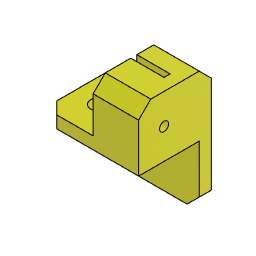
Z Belt Bottom Anchor Front_1x (Autodesk Fusion 360 design; units mm, degrees)
Autodesk Fusion 360 part; units mm, degrees
sketch "Sketch1" plane through (0, 0, 0) normal (0, 0, 1) x (1, 0, 0)
  line L0 (0, 0) -> (47, 0)
  line L1 (47, 0) -> (47, 20)
  line L2 (47, 20) -> (0, 20)
  line L3 (0, 20) -> (0, 0)
  line L4 (23.5, 20) -> (23.5, 0) construction
  line L5 (27, 20) -> (31, 20)
  line L6 (31, 20) -> (31, 0)
  line L7 (31, 0) -> (27, 0)
  line L8 (27, 0) -> (27, 20)
  line L9 (20, 20) -> (20, 0) construction
  dimension "d2" = 20
  dimension "d3" = 4
  dimension "d40" = 7
  dimension "d62" = 20
  constraint horizontal L0
  constraint vertical L1
  constraint horizontal L2
  constraint vertical L3
  constraint coincident L0.start L3.end
  constraint midpoint L2 L4.start
  constraint midpoint L0 L4.end
  constraint horizontal L5
  constraint vertical L6
  constraint horizontal L7
  constraint vertical L8
  constraint coincident L0 L6.end
  constraint coincident L2 L5.start
  constraint coincident L2 L9.start
  constraint coincident L0 L9.end
  constraint perpendicular L0 L9
  constraint symmetric L4 L5.start L9.start
  measures "d2" distance of L0.start L2.end
  measures "d3" distance of L5.start L5.end
  measures "d40" distance of L5.start L9.start
  measures "d62" distance of L0.start L9.end
extrude "Extrude1" add sketch "Sketch1" along normal blind 4 contours L0 L2 L3 L8 | L0 L2 L5 L6 L7 L8
extrude "Extrude2" add sketch "Sketch1" along normal blind 20 contours L0 L2 L5 L6 L7 L8
sketch "Sketch2" plane through (27, 0, 0) normal (-1, 0, 0) x (0, -1, 0)
  line L0 (-20, 4) -> (0, 4)
  line L1 (0, 4) -> (0, 20)
  line L2 (0, 20) -> (-20, 20)
  line L3 (-20, 20) -> (-20, 4)
  line L4 (-12.4, 14.4721) -> (-12.4, 20)
  line L5 (-14.4, 20) -> (-14.4, 10)
  circle A0 centre (-8.4, 10) radius 4
  line L6 (0, 12) -> (-8.4, 10) construction
  circle A1 centre (-8.4, 10) radius 6
  arc A2 (-12.4, 18.9443) -> (-9.0667, 15.9628) centre (-9.4, 18.9443) ccw
  circle A3 centre (-8.4, 10) radius 1.5
  circle A4 centre (-8.4, 10) radius 11.6 construction
  dimension "d45" = 2
  dimension "d48" = 12.4
  dimension "d52" = 3
  dimension "d63" = 12
  dimension "d64" = 2
  dimension "d65" = 2.5
  dimension "d66" = 4
  constraint coincident L2 L4.end
  constraint perpendicular L2 L4
  constraint coincident L2 L5.start
  constraint perpendicular L2 L5
  constraint midpoint L1 L6.start
  constraint coincident A0.centre L6
  constraint coincident A0.centre L6.end
  constraint concentric A0 A1
  constraint tangent L5 A1
  constraint coincident L5.end A1
  constraint coincident L4.start A1
  constraint tangent L4 A2
  constraint coincident A1 A2.end
  constraint coincident L4 A2.start
  constraint tangent A1 A2
  constraint tangent L0 A1
  constraint concentric A0 A3
  constraint concentric A0 A4
  constraint tangent L3 A4
  measures "d45" distance of L4.end L5.start
  measures "d48" distance of L1.end L4.end
  measures "d52" radius of A2
  measures "d63" diameter of A1
  measures "d64" distance of A0 A1
  measures "d65" distance of A0 A3
extrude "Extrude5" cut sketch "Sketch2" against normal blind 13 contours A3
extrude "Extrude3" add sketch "Sketch2" along normal blind 11 contours L0 L2 L3 L5 A1 | L0 L1 L2 L4 A1 A2 | A0
hole "Hole1" at (8, 10, 4) direction (0, 0, -1) diameter 5.5 depth 8 tip angle 118
sketch "Sketch4" plane through (0, 20, 0) normal (0, 1, 0) x (-1, 0, 0)
  line L0 (-31, 20) -> (-31, 0)
  line L1 (-31, 0) -> (0, 0)
  line L2 (0, 4) -> (-16, 4)
  line L3 (-16, 4) -> (-16, 20)
  line L4 (-31, 0) -> (-31, 20)
  line L5 (-16, 4) -> (-16, 20)
  line L6 (0, 4) -> (-16, 4)
  line L7 (0, 0) -> (-31, 0)
  line L8 (-16, 20) -> (-31, 20)
  line L9 (0, 0) -> (0, 4)
  line L10 (-31, 20) -> (-16, 20)
  line L11 (0, 0) -> (0, 4)
  line L12 (-31, 0) -> (0, 0)
  line L13 (0, 0) -> (0, -20)
  line L14 (0, -20) -> (-31, -20)
  line L15 (-31, -20) -> (-31, 0)
  dimension "d56" = 20
  constraint horizontal L12
  constraint vertical L13
  constraint horizontal L14
  constraint vertical L15
  constraint coincident L0.end L1.start
  constraint coincident L1.end L7.start
  measures "d56" distance of L0.end L14.end
extrude "Extrude4" add sketch "Sketch4" along normal blind 4
hole "Hole5" at (15.5, 20, -10) direction (0, 1, 0) diameter 5.5 depth 8 tip angle 118
chamfer "Chamfer5" distance 4 angle 45 5 edges at (23.5, 0, 20) (23.5, 24, 20) (0, 0, 2) (0, 22, -20) (31, 22, -20)
equation "d34 = 7 mm + 4 mm"
named bodies: "11mm Z Belt Bottom Anchor_1x_SN_BN"
